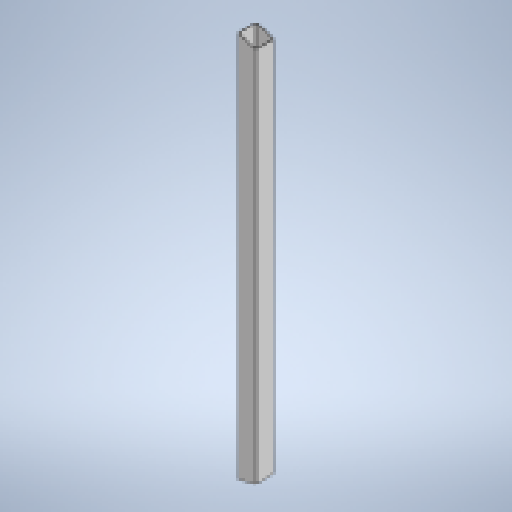
# Autodesk Inventor part: Crossbar
Saved by Autodesk Inventor 2025 (Build 290162010, 162A)
## iProperties
Created: 2024-07-03
Part Number: Crossbar
Material: Generic
Document SubType Name: Modeling
Designer: pokla
Density: 1 g/cm^3
Appearance: Default
Stock Number: Поперечина
Author: pokla
Autodesk Inventor part; units mm, degrees
ref_plane "YZ Plane" through (0, 0, 0) normal (1, 0, 0) x (0, 1, 0)
ref_plane "XZ Plane" through (0, 0, 0) normal (0, 1, 0) x (-1, 0, 0)
ref_plane "XY Plane" through (0, 0, 0) normal (0, 0, 1) x (1, 0, 0)
sketch "Sketch1" plane through (0, 0, 0) normal (0, 0, 1) x (1, 0, 0)
  line L0 (-60, -52) -> (-60, 52)
  line L1 (-52, 60) -> (52, 60)
  line L2 (60, 52) -> (60, -52)
  line L3 (52, -60) -> (-52, -60)
  arc A0 (-60, -52) -> (-52, -60) centre (-52, -52) ccw
  arc A1 (60, 52) -> (52, 60) centre (52, 52) ccw
  arc A2 (-52, 60) -> (-60, 52) centre (-52, 52) ccw
  arc A3 (52, -60) -> (60, -52) centre (52, -52) ccw
  arc A4 (-52, 56) -> (-56, 52) centre (-52, 52) ccw
  line L4 (-52, 56) -> (52, 56)
  arc A5 (56, 52) -> (52, 56) centre (52, 52) ccw
  line L5 (56, 52) -> (56, -52)
  arc A6 (52, -56) -> (56, -52) centre (52, -52) ccw
  line L6 (52, -56) -> (-52, -56)
  arc A7 (-56, -52) -> (-52, -56) centre (-52, -52) ccw
  line L7 (-56, -52) -> (-56, 52)
  point P0 (0, 0)
  point P1 (0, 0)
  point P2 (0, 60)
  point P3 (60, 0)
  dimension "d0" = 8
  dimension "d1" = 120
  dimension "d2" = 120
  dimension "d3" = 4
  constraints: 16 end point, 16 point on circle, 8 centre point, 8 tangent, 4 parallel, 3 equal radius, 2 coincident, 2 midpoint, 2 perpendicular, 1 horizontal, 1 horizontal alignment, 1 vertical alignment, 7 other
  measures "d0" radius of A0
  measures "d1" distance between parallel lines of L0 L2
  measures "d2" distance between parallel lines of L1 L3
  measures "d3" distance between parallel lines of L2 L5
extrude "Extrusion1" add sketch "Sketch1" along normal mid plane 2505
sketch "Sketch2" plane through (-52, -60, 1252.5) normal (0, -1, 0) x (1, 0, 0)
  line L0 (-8, -2505) -> (-8, 0) projected
  line L1 (-8, 0) -> (112, -32.1539)
  line L2 (112, -2505) -> (112, 0) projected
  line L3 (0, 0) -> (104, 0) projected
  line L4 (112, 0) -> (104, 0) projected
  line L5 (0, 0) -> (-8, 0) projected
  point P0 (52, -1252.5)
  dimension "d16" = 15
  constraints: 2 end point, 1 point on line
  measures "d16" angle of L3 L1
extrude "Extrusion2" cut sketch "Sketch2" against normal blind 2000
mirror "Mirror1" about plane through (0, 0, 0) normal (0, 0, 1) of "Extrusion2"
equation "\"d0\" = d6"
equation "\"d1\" = d7"
equation "\"d2\" = d8"
equation "\"d3\" = d9"
equation "\"d6\" = 8"
equation "\"d7\" = 120"
equation "\"d8\" = 120"
equation "\"d9\" = 4"
body "Solid1"
